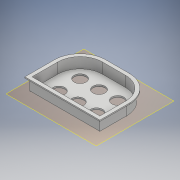
# Autodesk Inventor part: bottleHolder
Saved by Autodesk Inventor 2017 (Build 210142000, 142)
## iProperties
Created: 2016-11-02
Part Number: bottleHolder
Material: Generic
Document SubType Name: Modeling
Designer: Camilo
Density: 1 g/cm^3
Appearance: Default
Author: Camilo
Autodesk Inventor part; units mm, degrees
ref_plane "YZ Plane" through (0, 0, 0) normal (1, 0, 0) x (0, 1, 0)
ref_plane "XZ Plane" through (0, 0, 0) normal (0, 1, 0) x (-1, 0, 0)
ref_plane "XY Plane" through (0, 0, 0) normal (0, 0, 1) x (1, 0, 0)
ref_plane "Work Plane1" through (0, 0, -20) normal (0, 0, 1) x (1, 0, 0)
sketch "Sketch1" plane through (0, 0, -20) normal (0, 0, 1) x (1, 0, 0)
  arc A0 (-24.5816, 56) -> (-77, 3.5816) centre (-24.5816, 3.5816) ccw construction
  line L0 (-24.5816, 56) -> (24.5816, 56) construction
  arc A1 (77, 3.5816) -> (24.5816, 56) centre (24.5816, 3.5816) ccw construction
  line L1 (77, 3.5816) -> (77, -56) construction
  line L2 (77, -56) -> (-77, -56) construction
  line L3 (-77, -56) -> (-77, 3.5816) construction
  line L4 (87, 75) -> (-87, 75) construction
  line L5 (-87, 75) -> (-87, -75) construction
  line L6 (-87, -75) -> (87, -75) construction
  line L7 (87, -75) -> (87, 75) construction
  line L8 (24.5816, 53.5) -> (-24.5816, 53.5)
  arc A2 (-24.5816, 53.5) -> (-74.5, 3.5816) centre (-24.5816, 3.5816) ccw
  line L9 (-74.5, 3.5816) -> (-74.5, -53.5)
  line L10 (-74.5, -53.5) -> (74.5, -53.5)
  line L11 (74.5, -53.5) -> (74.5, 3.5816)
  arc A3 (74.5, 3.5816) -> (24.5816, 53.5) centre (24.5816, 3.5816) ccw
  point P0 (0, 0)
  dimension "d0" = 2.5
  constraints: 8 end point, 4 point on circle, 2 centre point, 5 other
  measures "d0" distance between parallel lines of L2 L10
extrude "Extrusion1" add sketch "Sketch1" along normal blind 5
sketch "Sketch2" plane through (0, 0, -15) normal (0, 0, 1) x (1, 0, 0)
  line L0 (24.5816, 53.5) -> (-24.5816, 53.5) projected
  arc A0 (-24.5816, 53.5) -> (-74.5, 3.5816) centre (-24.5816, 3.5816) ccw projected
  line L1 (-74.5, 3.5816) -> (-74.5, -53.5) projected
  line L2 (-74.5, -53.5) -> (74.5, -53.5) projected
  line L3 (74.5, -53.5) -> (74.5, 3.5816) projected
  arc A1 (74.5, 3.5816) -> (24.5816, 53.5) centre (24.5816, 3.5816) ccw projected
  line L4 (24.5816, 51) -> (-24.5816, 51)
  arc A2 (-24.5816, 51) -> (-72, 3.5816) centre (-24.5816, 3.5816) ccw
  line L5 (-72, 3.5816) -> (-72, -51)
  line L6 (-72, -51) -> (72, -51)
  line L7 (72, -51) -> (72, 3.5816)
  arc A3 (72, 3.5816) -> (24.5816, 51) centre (24.5816, 3.5816) ccw
  point P0 (0, 0)
  dimension "d3" = 2.5
  constraints: 8 end point, 4 point on circle, 2 centre point, 5 other
  measures "d3" distance between parallel lines of L2 L6
ref_plane "Work Plane2" through (-87, -75, 0) normal (0, 0, 1) x (1, 0, 0)
extrude "Extrusion2" add sketch "Sketch2" along normal up to surface (15 mm away)
sketch "Sketch3" plane through (-74.5, -53.5, 0) normal (0, 0, 1) x (1, 0, 0)
  arc A0 (146.5, 57.0816) -> (99.0816, 104.5) centre (99.0816, 57.0816) ccw projected
  line L0 (146.5, 2.5) -> (146.5, 57.0816) projected
  line L1 (2.5, 2.5) -> (146.5, 2.5) projected
  line L2 (2.5, 57.0816) -> (2.5, 2.5) projected
  arc A1 (49.9184, 104.5) -> (2.5, 57.0816) centre (49.9184, 57.0816) ccw projected
  line L3 (99.0816, 104.5) -> (49.9184, 104.5) projected
  arc A2 (149, 57.0816) -> (99.0816, 107) centre (99.0816, 57.0816) ccw projected
  line L4 (49.9184, 107) -> (99.0816, 107) projected
  arc A3 (49.9184, 107) -> (0, 57.0816) centre (49.9184, 57.0816) ccw projected
  line L5 (0, 0) -> (0, 57.0816) projected
  line L6 (149, 0) -> (0, 0) projected
  line L7 (149, 57.0816) -> (149, 0) projected
  point P0 (74.5, 53.5)
extrude "Extrusion3" add sketch "Sketch3" along normal blind 5
sketch "Sketch4" plane through (-74.5, -53.5, 5) normal (0, 0, 1) x (1, 0, 0)
  line L0 (146.5, 57.0816) -> (146.5, 2.5) projected
  line L1 (146.5, 2.5) -> (2.5, 2.5) projected
  line L2 (2.5, 2.5) -> (2.5, 57.0816) projected
  arc A0 (49.9184, 104.5) -> (2.5, 57.0816) centre (49.9184, 57.0816) ccw projected
  line L3 (49.9184, 104.5) -> (99.0816, 104.5) projected
  arc A1 (146.5, 57.0816) -> (99.0816, 104.5) centre (99.0816, 57.0816) ccw projected
  arc A2 (149, 57.0816) -> (99.0816, 107) centre (99.0816, 57.0816) ccw construction
  line L4 (99.0816, 107) -> (49.9184, 107) construction
  arc A3 (49.9184, 107) -> (0, 57.0816) centre (49.9184, 57.0816) ccw construction
  line L5 (0, 57.0816) -> (0, 0) construction
  line L6 (0, 0) -> (149, 0) construction
  line L7 (149, 0) -> (149, 57.0816) construction
  line L8 (154, -5) -> (-5, -5)
  line L9 (-5, -5) -> (-5, 57.0816)
  arc A4 (49.9184, 112) -> (-5, 57.0816) centre (49.9184, 57.0816) ccw
  line L10 (49.9184, 112) -> (99.0816, 112)
  arc A5 (154, 57.0816) -> (99.0816, 112) centre (99.0816, 57.0816) ccw
  line L11 (154, 57.0816) -> (154, -5)
  point P0 (74.5, 53.5)
  dimension "d8" = 5
  constraints: 8 end point, 4 point on circle, 2 centre point, 5 other
  measures "d8" distance between parallel lines of L8 L6
extrude "Extrusion4" add sketch "Sketch4" along normal blind 2.5
chamfer "Chamfer1" distance 5 angle 45 6 edges at (-74.5, -24.9592, 5) (-59.8792, 38.8792, 5) (0, 53.5, 5) (59.8792, 38.8792, 5) (74.5, -24.9592, 5) (0, -53.5, 5)
sketch "Sketch5" plane through (0, 0, -15) normal (0, 0, 1) x (1, 0, 0)
  circle A0 centre (-40, -26) radius 12.75
  line L0 (-72, 3.5816) -> (-72, -51) projected
  line L1 (-72, -51) -> (72, -51) projected
  line L2 (72, -51) -> (72, 3.5816) projected
  arc A1 (72, 3.5816) -> (24.5816, 51) centre (24.5816, 3.5816) ccw projected
  line L3 (24.5816, 51) -> (-24.5816, 51) projected
  arc A2 (-24.5816, 51) -> (-72, 3.5816) centre (-24.5816, 3.5816) ccw projected
  circle A3 centre (-40, 19) radius 12.75
  circle A4 centre (0, -26) radius 12.75
  circle A5 centre (0, 19) radius 12.75
  circle A6 centre (40, -26) radius 12.75
  circle A7 centre (40, 19) radius 12.75
  point P0 (0, 0)
  dimension "d14" = 25.5
  dimension "d15" = 25
  dimension "d16" = 32
  dimension "d19" = 45
  dimension "d22" = 40
  constraints: 6 centre point, 1 horizontal, 1 vertical, 10 other
  measures "d14" diameter of A0
  measures "d15" distance from line of L1 A0.centre
  measures "d16" distance from line of A0.centre L0
  measures "d19" distance of A0.centre A3.centre
  measures "d22" distance of A0.centre A4.centre
extrude "Extrusion5" cut sketch "Sketch5" against normal through all contours A0 | A3 | A4 | A5 | A6 | A7
fillet "Fillet1" radius 2 6 edges at (27.25, -26, -20) (27.25, 19, -20) (-12.75, -26, -20) (-12.75, 19, -20) (-52.75, -26, -20) (-52.75, 19, -20)
fillet "Fillet2" radius 2 6 edges at (59.8792, 38.8792, -20) (0, 53.5, -20) (-59.8792, 38.8792, -20) (-74.5, -24.9592, -20) (74.5, -24.9592, -20) (0, -53.5, -20)
body "Solid1"
